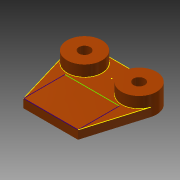
# Autodesk Inventor part: BED TENSIONER MOUNT
Saved by Autodesk Inventor 2013 (Build 170138000, 138)
## iProperties
Created: 2014-06-23
Part Number: BED TENSIONER MOUNT
Material: Generic
Document SubType Name: Modeling
Designer: employee
Density: 1 g/cm^3
Author: employee
Autodesk Inventor part; units mm, degrees
ref_plane "YZ Plane" through (0, 0, 0) normal (1, 0, 0) x (0, 1, 0)
ref_plane "XZ Plane" through (0, 0, 0) normal (0, 1, 0) x (-1, 0, 0)
ref_plane "XY Plane" through (0, 0, 0) normal (0, 0, 1) x (1, 0, 0)
sketch "Sketch1" plane through (0, 0, 0) normal (0, 0, 1) x (1, 0, 0)
  line L0 (-12.5, 0) -> (12.5, 0)
  circle A0 centre (-12.5, 0) radius 8
  circle A1 centre (12.5, 0) radius 8
  circle A2 centre (-12.5, 0) radius 2.6
  circle A3 centre (12.5, 0) radius 2.6
  line L1 (-12.5, -8) -> (12.5, -8)
  line L2 (12.5, -8) -> (12.5, -28)
  line L3 (12.5, -28) -> (-12.5, -28)
  line L4 (-12.5, -28) -> (-12.5, -8)
  line L5 (-12.5, -28) -> (-20.1665, -2.2857)
  line L6 (12.5, -28) -> (20.1665, -2.2857)
  line L7 (12.5, 8) -> (-12.5, 8)
  point P0 (0, 0)
  point P1 (0, 0)
  point P2 (19.726, -3.4329)
  point P3 (0, -8)
  dimension "d0" = 16
  dimension "d2" = 25
  dimension "d3" = 5.2
  dimension "d44" = 20
  dimension "d45" = 25
  constraints: 16 end point, 5 coincident, 5 point on circle, 5 tangent, 4 centre point, 2 equal radius, 2 horizontal, 2 midpoint, 2 parallel, 1 perpendicular, 1 vertical alignment
  measures "d0" diameter of A0
  measures "d2" distance of L0.start L0.end
  measures "d3" diameter of A2
  measures "d44" distance of L1.end L2.end
  measures "d45" distance of L2.end L3.end
extrude "Extrusion1" add sketch "Sketch1" along normal blind 4
sketch "Sketch12" plane through (0, 0, 4) normal (0, 0, 1) x (1, 0, 0)
  circle A0 centre (12.5, 0) radius 2.6 projected
  circle A1 centre (-12.5, 0) radius 2.6 projected
  arc A2 (-12.5, 8) -> (-20.1665, -2.2857) centre (-12.5, 0) ccw projected
  arc A3 (20.1665, -2.2857) -> (12.5, 8) centre (12.5, 0) ccw projected
  circle A4 centre (-12.5, 0) radius 8
  circle A5 centre (12.5, 0) radius 8
  point P0 (0, 0)
  constraints: 2 coincident, 2 vertical alignment, 4 other
extrude "Extrusion10" add sketch "Sketch12" along normal blind 5
sketch "Sketch13" plane through (0, 0, 4) normal (0, 0, 1) x (1, 0, 0)
  line L0 (12.5, -28) -> (-12.5, -28)
  line L1 (-12.5, -28) -> (-12.5, -8)
  line L2 (-12.5, -8) -> (12.5, -8)
  line L3 (12.5, -8) -> (12.5, -28)
  circle A0 centre (-12.5, 0) radius 8 projected
  point P0 (0, 0)
  constraints: 8 end point, 2 parallel, 1 horizontal, 1 perpendicular, 1 tangent
extrude "Extrusion11" add sketch "Sketch13" along normal blind 26 contours L0 L1 L2 L3
sketch "Sketch14" plane through (0, 0, 0) normal (0, 0, -1) x (-1, 0, 0)
  line L0 (-12.5, 8) -> (12.5, 8) projected
  line L1 (12.5, -28) -> (-12.5, -28) projected
  line L2 (-8, 8) -> (-8, -28)
  line L3 (8, 8) -> (8, -28)
  point P0 (0, 0)
  dimension "d50" = 8
  dimension "d51" = 8
  constraints: 4 end point, 4 point on line, 1 parallel, 1 perpendicular
  measures "d50" distance from line of L3 point (0, 0)
  measures "d51" distance from line of L2 point (0, 0)
extrude "Extrusion12" cut sketch "Sketch14" against normal blind 15
sketch "Sketch16" plane through (0, 0, 0) normal (0, 0, -1) x (-1, 0, 0)
  circle A0 centre (-12.5, 0) radius 2.6 projected
  line L0 (-8, -28) -> (-8, 8) projected
  line L1 (-12.5, 8) -> (-8, 8) projected
  arc A1 (-12.5, 8) -> (-20.1665, -2.2857) centre (-12.5, 0) ccw projected
  line L2 (-12.5, -28) -> (-20.1665, -2.2857) projected
  line L3 (-8, -28) -> (-12.5, -28) projected
  line L4 (-8, 8) -> (8, 8)
  line L5 (8, 8) -> (8, -28)
  line L6 (8, -28) -> (-8, -28)
  line L7 (-8, -28) -> (-8, 8)
  point P0 (0, 0)
  constraints: 8 end point, 2 parallel, 1 horizontal, 1 perpendicular
extrude "Extrusion13" add sketch "Sketch16" against normal blind 4 contours L0 L4 L5 L6
sketch "Sketch17" plane through (0, 0, 4) normal (0, 0, 1) x (1, 0, 0)
  arc A0 (12.5, 8) -> (8, 6.6144) centre (12.5, 0) ccw projected
  arc A1 (-8, 6.6144) -> (-12.5, 8) centre (-12.5, 0) ccw projected
  line L0 (-8, -6.6144) -> (-8, 6.6144) projected
  arc A2 (-12.5, -8) -> (-8, -6.6144) centre (-12.5, 0) ccw projected
  line L1 (-12.5, -8) -> (-8, -8) projected
  line L2 (-8, -28) -> (-8, -8) projected
  line L3 (8, -8) -> (8, -28) projected
  line L4 (8, -8) -> (12.5, -8) projected
  arc A3 (8, -6.6144) -> (12.5, -8) centre (12.5, 0) ccw projected
  line L5 (8, 6.6144) -> (8, -6.6144) projected
  line L6 (-12.5, -28) -> (-12.5, -8) projected
  arc A4 (-20.1665, -2.2857) -> (-12.5, -8) centre (-12.5, 0) ccw projected
  line L7 (-20.1665, -2.2857) -> (-12.5, -28) projected
  line L8 (12.5, -8) -> (12.5, -28) projected
  line L9 (12.5, -28) -> (20.1665, -2.2857) projected
  arc A5 (12.5, -8) -> (20.1665, -2.2857) centre (12.5, 0) ccw projected
  arc A6 (-6.25, -4.9937) -> (-8, 6.6144) centre (-12.5, 0) ccw
  arc A7 (-6.25, -4.9937) -> (-8, -9.9875) centre (0, -9.9875) ccw
  arc A8 (8, 6.6144) -> (6.25, -4.9937) centre (12.5, 0) ccw
  arc A9 (8, -9.9875) -> (6.25, -4.9937) centre (0, -9.9875) ccw
  point P0 (0, 0)
  constraints: 8 point on circle, 6 tangent, 4 centre point, 2 concentric, 2 equal radius, 2 point on line
extrude "Extrusion14" add sketch "Sketch17" along normal blind 5
sketch "Sketch18" plane through (0, 0, 30) normal (0, 0, 1) x (1, 0, 0)
  line L0 (-12.5, -28) -> (12.5, -28) projected
  line L1 (-12.5, -8) -> (-12.5, -28) projected
  circle A0 centre (0, -20) radius 5.08
  line L2 (-7.633, -12.367) -> (7.633, -12.367)
  circle A1 centre (-7.633, -12.367) radius 1
  circle A2 centre (7.633, -12.367) radius 1
  point P0 (0, 0)
  point P1 (0, -28)
  point P2 (0, -12.367)
  dimension "d58" = 10.16
  dimension "d60" = 8
  dimension "d61" = 2
  dimension "d62" = 7.633
  dimension "d63" = 7.633
  constraints: 3 centre point, 2 coincident, 2 end point, 2 midpoint, 2 vertical alignment, 1 equal radius, 1 perpendicular
  measures "d58" diameter of A0
  measures "d60" distance from line of A0.centre L0
  measures "d61" diameter of A2
  measures "d62" distance of point (0, -12.367) A0.centre
  measures "d63" horizontal distance of L2.start A0.centre
extrude "Extrusion15" cut sketch "Sketch18" against normal blind 15
sketch "Sketch19" plane through (0, 0, 0) normal (0, 0, -1) x (-1, 0, 0)
  line L0 (12.5, -28) -> (-12.5, -28) projected
  circle A0 centre (0, -20) radius 5.08 projected
  circle A1 centre (0, -20) radius 8
  point P0 (0, 0)
  constraints: 1 centre point, 1 coincident, 1 tangent
extrude "Extrusion16" cut sketch "Sketch19" against normal up to surface (4 mm away) contours A0 | A1
sketch "Sketch20" plane through (0, 0, 4) normal (0, 0, 1) x (1, 0, 0)
  arc A0 (-8, -20) -> (0, -28) centre (0, -20) ccw projected
  line L0 (-8, -28) -> (-8, -20) projected
  line L1 (-8, -28) -> (0, -28) projected
  arc A1 (0, -28) -> (8, -20) centre (0, -20) ccw projected
  line L2 (0, -28) -> (8, -28) projected
  line L3 (8, -20) -> (8, -28) projected
  point P0 (0, 0)
extrude "Extrusion17" cut sketch "Sketch20" against normal through all
ref_plane "Work Plane1" through (0, 0, 6.5) normal (0, 0, 1) x (1, 0, 0)
sketch "Sketch21" plane through (0, 0, 6.5) normal (0, 0, 1) x (1, 0, 0)
  arc A0 (8, -9.9875) -> (6.25, -4.9937) centre (0, -9.9875) ccw projected
  arc A1 (20.1665, -2.2857) -> (6.25, -4.9937) centre (12.5, 0) ccw projected
  line L0 (20.1665, -2.2857) -> (12.5, -28) projected
  line L1 (12.5, -28) -> (8, -28) construction
  line L2 (8, -28) -> (8, -9.9875) projected
  arc A2 (-6.25, -4.9937) -> (-8, -9.9875) centre (0, -9.9875) ccw projected
  line L3 (-8, -9.9875) -> (-8, -28) projected
  line L4 (-8, -28) -> (-12.5, -28) construction
  line L5 (-12.5, -28) -> (-20.1665, -2.2857) projected
  arc A3 (-6.25, -4.9937) -> (-20.1665, -2.2857) centre (-12.5, 0) ccw projected
  circle A4 centre (12.5, 0) radius 2.6 projected
  circle A5 centre (-12.5, 0) radius 2.6 projected
  point P0 (0, 0)
sketch "Sketch22" plane through (-12.5, -28, 30) normal (0, -1, 0) x (1, 0, 0)
  line L0 (4.5, -30) -> (4.5, -15) projected
  line L1 (0, -30) -> (4.5, -30) projected
  line L2 (4.5, -22.5) -> (4, -23.5)
  line L3 (4, -23.5) -> (4.5, -24.5)
  line L4 (4.5, -22.5) -> (4.5, -24.5)
  point P0 (12.5, -30)
  point P1 (4.5, -23.5)
  point P2 (4.5, -23.5)
  point P3 (4.5, -23.5)
  dimension "d71" = 0.5
  dimension "d73" = 2
  constraints: 6 end point, 2 midpoint, 1 coincident, 1 equal length, 1 perpendicular, 1 point on line
  measures "d71" distance of point (4.5, -23.5) L2.end
  measures "d73" distance of L2.start L3.end
sweep "Sweep1" cut profiles "Sketch22" path "Sketch21" path curves L3 A2 A3 L5
sketch "Sketch23" plane through (-12.5, -28, 7.5) normal (-0.2857143, 0.9583148, 0) x (0.9583148, 0.2857143, 0)
  line L0 (0.5, 1) -> (0, 2) projected
  line L1 (0, 2) -> (0, 0) projected
  line L2 (0, 0) -> (0.5, 1) projected
  point P0 (19.9789, 7.5)
extrude "Extrusion18" cut sketch "Sketch23" against normal through all
mirror "Mirror2" about plane through (0, 0, 0) normal (1, 0, 0) of "Sweep1", "Extrusion18"
body "Solid1"
